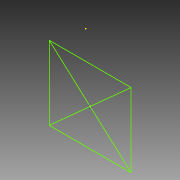
# Autodesk Inventor part: Ruler
Saved by Autodesk Inventor 2012 SP2 (Build 160219200, 219)
## iProperties
Created: 2014-02-09
Part Number: Ruler
Material: Default
Document SubType Name: Modeling
Designer: 1
Density: 1 g/cm^3
Author: 1
Autodesk Inventor part; units mm, degrees
ref_plane "YZ Plane" through (0, 0, 0) normal (1, 0, 0) x (0, 1, 0)
ref_plane "XZ Plane" through (0, 0, 0) normal (0, 1, 0) x (-1, 0, 0)
ref_plane "XY Plane" through (0, 0, 0) normal (0, 0, 1) x (1, 0, 0)
sketch "Sketch1" plane through (0, 0, 0) normal (0, 0, 1) x (1, 0, 0)
  line L0 (178.3811, -162.3451) -> (-127.8103, -162.3451)
  line L1 (-127.8103, -162.3451) -> (-127.8103, -582.0869)
  line L2 (-127.8103, -582.0869) -> (178.3811, -582.0869)
  line L3 (178.3811, -582.0869) -> (178.3811, -162.3451)
  circle A0 centre (25.2854, -372.216) radius 2.2409 projected
  line L4 (178.3811, -162.3451) -> (-127.8103, -582.0869)
  line L5 (178.3811, -582.0869) -> (-127.8103, -162.3451)
  point P0 (0, 0)
  constraints: 12 end point, 2 midpoint, 2 parallel, 1 coincident, 1 horizontal, 1 perpendicular
extrude "Extrusion1" add sketch "Sketch1" along normal blind 19.05
sketch "Sketch2" plane through (0, 0, 19.05) normal (0, 0, 1) x (1, 0, 0)
  line L0 (178.3811, -582.0869) -> (-127.8103, -582.0869) projected
  line L1 (-127.8103, -162.3451) -> (178.3811, -162.3451) projected
  line L2 (-10.8645, -162.3451) -> (-10.8645, -582.0869)
  circle A0 centre (25.2854, -372.216) radius 4.386 projected
  line L3 (61.4353, -582.0869) -> (61.4353, -162.3451)
  line L4 (-10.8645, -162.3451) -> (61.4353, -582.0869)
  line L5 (61.4353, -162.3451) -> (-10.8645, -582.0869)
  line L6 (-10.8645, -162.3451) -> (61.4353, -162.3451)
  line L7 (61.4353, -582.0869) -> (-10.8645, -582.0869)
  point P0 (0, 0)
  point P1 (25.2854, -372.216)
  constraints: 12 end point, 4 point on line, 2 collinear, 2 perpendicular, 1 coincident, 1 midpoint
extrude "Extrusion2" add sketch "Sketch2" along normal blind 11.1125
sketch "Sketch3" plane through (0, 0, 30.1625) normal (0, 0, 1) x (1, 0, 0)
  line L0 (-10.8645, -582.0869) -> (-10.8645, -162.3451) projected
  line L1 (61.4353, -162.3451) -> (61.4353, -582.0869) projected
  circle A0 centre (25.2854, -372.216) radius 4.386 projected
  line L2 (-10.8645, -203.9512) -> (61.4353, -203.9512)
  line L3 (61.4353, -203.9512) -> (61.4353, -208.4802)
  line L4 (61.4353, -208.4802) -> (-10.8645, -208.4802)
  line L5 (-10.8645, -208.4802) -> (-10.8645, -203.9512)
  line L6 (-10.8645, -216.6512) -> (61.4353, -216.6512)
  line L7 (61.4353, -216.6512) -> (61.4353, -221.1802)
  line L8 (61.4353, -221.1802) -> (-10.8645, -221.1802)
  line L9 (-10.8645, -221.1802) -> (-10.8645, -216.6512)
  line L10 (25.2854, -372.216) -> (-128.4851, -372.216) construction
  line L11 (-10.8645, -540.4809) -> (61.4353, -540.4809)
  line L12 (61.4353, -540.4809) -> (61.4353, -535.9519)
  line L13 (61.4353, -535.9519) -> (-10.8645, -535.9519)
  line L14 (-10.8645, -535.9519) -> (-10.8645, -540.4809)
  line L15 (61.4353, -527.7809) -> (61.4353, -523.2519)
  line L16 (-10.8645, -523.2519) -> (-10.8645, -527.7809)
  line L17 (-10.8645, -527.7809) -> (61.4353, -527.7809)
  line L18 (61.4353, -523.2519) -> (-10.8645, -523.2519)
  point P0 (0, 0)
  dimension "d6" = 12.7
  constraints: 34 end point, 8 symmetric about line, 3 parallel, 2 collinear, 1 horizontal, 1 perpendicular, 1 point on line, 1 vertical, 8 other
  measures "d6" distance of L2.end L7.start
extrude "Extrusion3" add sketch "Sketch3" along normal blind 19.05 contours L0 L13 L1 L11 | L0 L18 L1 L17 | L0 L6 L1 L8 | L0 L2 L1 L4
fillet "Fillet1" radius 17.4625 4 edges at (-127.8103, -582.0869, 9.525) (-127.8103, -162.3451, 9.525) (178.3811, -582.0869, 9.525) (178.3811, -162.3451, 9.525)
sketch "Sketch4" plane through (-10.8645, -582.0869, 19.05) normal (-1, 0, 0) x (0, 0, 1)
  line L0 (11.1125, 0) -> (11.1125, 41.606) projected
  line L1 (11.1125, 41.606) -> (30.1625, 41.606) projected
  line L2 (30.1625, 41.606) -> (30.1625, 46.135) projected
  line L3 (11.1125, 46.135) -> (30.1625, 46.135) projected
  line L4 (11.1125, 54.306) -> (30.1625, 54.306) projected
  line L5 (30.1625, 54.306) -> (30.1625, 58.835) projected
  line L6 (11.1125, 58.835) -> (30.1625, 58.835) projected
  line L7 (11.1125, 58.835) -> (11.1125, 360.9067) projected
  line L8 (11.1125, 360.9067) -> (30.1625, 360.9067) projected
  line L9 (30.1625, 360.9067) -> (30.1625, 365.4357) projected
  line L10 (11.1125, 365.4357) -> (30.1625, 365.4357) projected
  line L11 (11.1125, 373.6067) -> (30.1625, 373.6067) projected
  line L12 (30.1625, 373.6067) -> (30.1625, 378.1357) projected
  line L13 (11.1125, 378.1357) -> (30.1625, 378.1357) projected
  line L14 (0, 0) -> (0, 419.7418) projected
  line L15 (0, 0) -> (11.1125, 0) projected
  line L16 (11.1125, 378.1357) -> (3.1565, 378.1357)
  line L17 (3.1565, 378.1357) -> (3.1565, 373.6067)
  line L18 (3.1565, 373.6067) -> (11.1125, 373.6067)
  line L19 (11.1125, 365.4357) -> (3.1565, 365.4357)
  line L20 (3.1565, 365.4357) -> (3.1565, 360.9067)
  line L21 (3.1565, 360.9067) -> (11.1125, 360.9067)
  line L22 (11.1125, 58.835) -> (3.1565, 58.835)
  line L23 (3.1565, 58.835) -> (3.1565, 54.306)
  line L24 (3.1565, 54.306) -> (11.1125, 54.306)
  line L25 (11.1125, 46.135) -> (3.1565, 46.135)
  line L26 (3.1565, 46.135) -> (3.1565, 41.606)
  line L27 (3.1565, 41.606) -> (11.1125, 41.606)
  point P0 (-19.05, 582.0869)
  constraints: 24 end point, 5 parallel, 5 perpendicular
extrude "Extrusion4" add sketch "Sketch4" along normal blind 6.35
sketch "Sketch5" plane through (-10.8645, -582.0869, 30.1625) normal (0, -1, 0) x (1, 0, 0)
  line L0 (0, 0) -> (72.2998, 0)
  line L1 (72.2998, 0) -> (72.2998, -11.1125)
  line L2 (72.2998, -11.1125) -> (0, -11.1125)
  line L3 (0, -11.1125) -> (0, 0)
  point P0 (10.8645, -30.1625)
  constraints: 8 end point, 2 parallel, 1 horizontal, 1 perpendicular
extrude "Extrusion5" add sketch "Sketch5" along normal blind 19.05
sketch "Sketch6" plane through (-10.8645, -162.3451, 30.1625) normal (0, 1, 0) x (1, 0, 0)
  line L0 (0, 11.1125) -> (72.2998, 11.1125)
  line L1 (72.2998, 11.1125) -> (72.2998, 0)
  line L2 (72.2998, 0) -> (0, 0)
  line L3 (0, 0) -> (0, 11.1125)
  point P0 (10.8645, 30.1625)
  constraints: 8 end point, 2 parallel, 1 horizontal, 1 perpendicular
extrude "Extrusion6" add sketch "Sketch6" along normal blind 6.35
body "Solid1"
